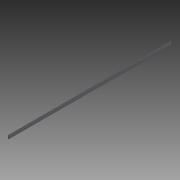
# Autodesk Inventor part: X_Rai-SquareBar-Rev3
Saved by Autodesk Inventor 2015 (Build 190159000, 159)
## iProperties
Created: 2017-01-08
Part Number: X_Rai-SquareBar-Rev3
Material: Generic
Document SubType Name: Modeling
Designer: Guy
Density: 1 g/cm^3
Appearance: Default
Author: Guy
Autodesk Inventor part; units mm, degrees
ref_plane "YZ Plane" through (0, 0, 0) normal (1, 0, 0) x (0, 1, 0)
ref_plane "XZ Plane" through (0, 0, 0) normal (0, 1, 0) x (-1, 0, 0)
ref_plane "XY Plane" through (0, 0, 0) normal (0, 0, 1) x (1, 0, 0)
sketch "Sketch1" plane through (0, 0, 0) normal (0, 0, 1) x (1, 0, 0)
  line L0 (0, 0) -> (6.35, 0)
  line L1 (6.35, 0) -> (6.35, 38.1)
  line L2 (6.35, 38.1) -> (0, 38.1)
  line L3 (0, 38.1) -> (0, 0)
  dimension "d0" = 6.35
  dimension "d1" = 38.1
  constraints: 8 end point, 2 parallel, 1 horizontal, 1 perpendicular
  measures "d0" distance between parallel lines of L3 L1
  measures "d1" distance between parallel lines of L0 L2
extrude "Extrusion1" add sketch "Sketch1" along normal blind 2000
sketch "Sketch2" plane through (6.35, 38.1, 2000) normal (1, 0, 0) x (0, 0, -1)
  line L0 (2000, -38.1) -> (2000, 0) projected
  line L1 (2000, 0) -> (0, 0) projected
  line L2 (0, -38.1) -> (0, 0) projected
  line L3 (2000, -38.1) -> (0, -38.1) projected
  circle A0 centre (200, -19.05) radius 4
  circle A1 centre (400, -19.05) radius 4
  circle A2 centre (600, -19.05) radius 4
  circle A3 centre (1400, -19.05) radius 4
  circle A4 centre (1600, -19.05) radius 4
  circle A5 centre (1800, -19.05) radius 4
  dimension "d4" = 8
  dimension "d5" = 19.05
  dimension "d6" = 8
  dimension "d7" = 8
  dimension "d8" = 8
  dimension "d9" = 8
  dimension "d10" = 8
  dimension "d11" = 200
  dimension "d12" = 200
  dimension "d13" = 200
  dimension "d14" = 200
  dimension "d15" = 200
  dimension "d16" = 200
  dimension "d17" = 19.05
  dimension "d18" = 19.05
  dimension "d19" = 19.05
  dimension "d20" = 19.05
  dimension "d21" = 19.05
  constraints: 6 centre point
  measures "d4" diameter of A0
  measures "d5" distance from line of L3 A0.centre
  measures "d6" diameter of A1
  measures "d7" diameter of A2
  measures "d8" diameter of A3
  measures "d9" diameter of A4
  measures "d10" diameter of A5
  measures "d11" distance from line of A0.centre L2
  measures "d12" distance of A0.centre A1.centre
  measures "d13" distance of A1.centre A2.centre
  measures "d14" distance from line of L0 A5.centre
  measures "d15" distance of A4.centre A5.centre
  measures "d16" distance of A3.centre A4.centre
  measures "d17" distance from line of L3 A1.centre
  measures "d18" distance from line of L3 A2.centre
  measures "d19" distance from line of A3.centre L3
  measures "d20" distance from line of L3 A4.centre
  measures "d21" distance from line of L3 A5.centre
extrude "Extrusion3" cut sketch "Sketch2" against normal blind 10 contours A0 | A1 | A2 | A3 | A4 | A5
body "Solid1"
